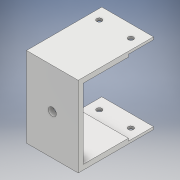
# Autodesk Inventor part: Forearm2 v2
Saved by Autodesk Inventor 2018 (Build 220112000, 112)
## iProperties
Created: 2018-04-13
Part Number: Forearm2 v2
Material: Plastique ABS
Document SubType Name: Modeling
Designer: Thomas
Density: 1.06 g/cm^3
Appearance: Lisse - Blanc
Author: Thomas
Autodesk Inventor part; units mm, degrees
ref_plane "YZ Plane" through (0, 0, 0) normal (1, 0, 0) x (0, 1, 0)
ref_plane "XZ Plane" through (0, 0, 0) normal (0, 1, 0) x (-1, 0, 0)
ref_plane "XY Plane" through (0, 0, 0) normal (0, 0, 1) x (1, 0, 0)
sketch "Esquisse1" plane through (0, 0, 0) normal (0, 0, 1) x (1, 0, 0)
  line L0 (0, 0) -> (51.5, 0)
  line L1 (51.5, 0) -> (51.5, -75)
  line L2 (51.5, -75) -> (0, -75)
  line L3 (0, -75) -> (0, 0)
  dimension "d0" = 51.5
  dimension "d1" = 75
  constraints: 8 end point, 2 parallel, 1 horizontal, 1 perpendicular
  measures "d0" distance of L0.start L0.end
  measures "d1" distance of L0.end L1.end
extrude "Extrusion1" add sketch "Esquisse1" along normal blind 5
sketch "Esquisse2" plane through (0, 0, 5) normal (0, 0, 1) x (1, 0, 0)
  line L0 (0, 0) -> (51.5, 0)
  line L1 (51.5, 0) -> (51.5, -25)
  line L2 (51.5, -25) -> (0, -25)
  line L3 (0, -25) -> (0, 0)
  dimension "d4" = 25
  constraints: 8 end point, 2 parallel, 1 horizontal, 1 perpendicular
  measures "d4" distance of L2.end L0.start
extrude "Extrusion2" cut sketch "Esquisse2" against normal blind 2.5
sketch "Esquisse3" plane through (0, 0, 2.5) normal (0, 0, 1) x (1, 0, 0)
  circle A0 centre (10, -12.5) radius 2.6
  circle A1 centre (41.5, -12.5) radius 2.6
  line L0 (0, 0) -> (51.5, 0) projected
  line L1 (0, -25) -> (0, 0) projected
  line L2 (51.5, 0) -> (51.5, -25) projected
  dimension "d7" = 5.2
  dimension "d8" = 5.2
  dimension "d9" = 12.5
  dimension "d10" = 10
  dimension "d11" = 12.5
  dimension "d12" = 10
  constraints: 2 centre point
  measures "d7" diameter of A0
  measures "d8" diameter of A1
  measures "d9" distance from line of L0 A0.centre
  measures "d10" distance from line of L1 A0.centre
  measures "d11" distance from line of L0 A1.centre
  measures "d12" distance from line of L2 A1.centre
extrude "Extrusion3" cut sketch "Esquisse3" against normal blind 2.5
sketch "Esquisse4" plane through (0, 0, 5) normal (0, 0, 1) x (1, 0, 0)
  line L0 (0, -75) -> (51.5, -75)
  line L1 (51.5, -75) -> (51.5, -70)
  line L2 (51.5, -70) -> (0, -70)
  line L3 (0, -70) -> (0, -75)
  dimension "d15" = 5
  constraints: 8 end point, 2 parallel, 1 horizontal, 1 perpendicular
  measures "d15" distance of L0.end L1.end
extrude "Extrusion4" add sketch "Esquisse4" along normal blind 70
sketch "Esquisse6" plane through (0, -75, 0) normal (0, -1, 0) x (1, 0, 0)
  line L0 (51.5, 5) -> (51.5, 75) projected
  line L1 (51.5, 75) -> (0, 75)
  line L2 (0, 75) -> (0, 80)
  line L3 (0, 80) -> (51.5, 80)
  line L4 (51.5, 80) -> (51.5, 75)
  point P0 (0, 0)
  dimension "d19" = 5
  constraints: 8 end point, 2 parallel, 1 horizontal, 1 perpendicular
  measures "d19" distance of L3.end L0.end
extrude "Extrusion5" add sketch "Esquisse6" against normal blind 75
sketch "Esquisse7" plane through (51.5, -70, 75) normal (0, 0, -1) x (-1, 0, 0)
  line L0 (0, 70) -> (51.5, 70) projected
  line L1 (0, 70) -> (51.5, 70)
  line L2 (51.5, 70) -> (51.5, 45)
  line L3 (51.5, 45) -> (0, 45)
  line L4 (0, 45) -> (0, 70)
  dimension "d22" = 25
  constraints: 8 end point, 2 parallel, 1 horizontal, 1 perpendicular
  measures "d22" distance of L1.end L2.end
extrude "Extrusion6" cut sketch "Esquisse7" against normal blind 2.5
sketch "Esquisse8" plane through (51.5, -70, 77.5) normal (0, 0, -1) x (-1, 0, 0)
  circle A0 centre (10, 57.5) radius 2.6
  circle A1 centre (41.5, 57.5) radius 2.6
  line L0 (0, 45) -> (0, 70) projected
  line L1 (51.5, 70) -> (51.5, 45) projected
  line L2 (0, 70) -> (51.5, 70) projected
  dimension "d25" = 5.2
  dimension "d26" = 5.2
  dimension "d27" = 10
  dimension "d28" = 10
  dimension "d29" = 12.5
  dimension "d30" = 12.5
  constraints: 2 centre point
  measures "d25" diameter of A0
  measures "d26" diameter of A1
  measures "d27" distance from line of L0 A0.centre
  measures "d28" distance from line of L1 A1.centre
  measures "d29" distance from line of L2 A0.centre
  measures "d30" distance from line of L2 A1.centre
extrude "Extrusion7" cut sketch "Esquisse8" against normal blind 2.5
sketch "Esquisse9" plane through (0, -75, 0) normal (0, -1, 0) x (1, 0, 0)
  line L0 (0, 80) -> (51.5, 80) construction
  line L1 (51.5, 0) -> (51.5, 2.5) construction
  line L2 (0, 80) -> (51.5, 0) construction
  line L3 (51.5, 80) -> (0, 0) construction
  circle A0 centre (25.75, 40) radius 4
  dimension "d33" = 8
  constraints: 4 end point, 1 centre point, 1 midpoint
  measures "d33" diameter of A0
extrude "Extrusion8" cut sketch "Esquisse9" against normal blind 5
